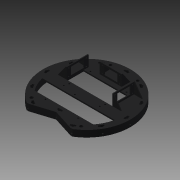
# Autodesk Inventor part: Middle Plate
Saved by Autodesk Inventor 2015 (Build 190159000, 159)
## iProperties
Created: 2015-10-10
Part Number: Middle Plate
Material: ABS Plastic
Document SubType Name: Modeling
Designer: James
Density: 1.06 g/cm^3
Appearance: Smooth - White
Mass: 170.874 g
Surface Area: 729.36 cm^2
Volume: 161.202 cm^3
Author: James
Autodesk Inventor part; units mm, degrees
ref_plane "YZ Plane" through (0, 0, 0) normal (1, 0, 0) x (0, 1, 0)
ref_plane "XZ Plane" through (0, 0, 0) normal (0, 1, 0) x (-1, 0, 0)
ref_plane "XY Plane" through (0, 0, 0) normal (0, 0, 1) x (1, 0, 0)
sketch "Sketch1" plane through (0, 0, 0) normal (0, 1, 0) x (-1, 0, 0)
  line L0 (70, 0) -> (70, 48.2183)
  line L1 (70, 0) -> (70, -48.2183)
  arc A0 (70, 48.2183) -> (70, -48.2183) centre (0, 0) ccw
  arc A1 (85, 52.6783) -> (85, -52.6783) centre (0, 0) ccw
  line L2 (85, -52.6783) -> (85, -47.6783)
  line L3 (85, 52.6783) -> (85, 47.6783)
  line L4 (85, -47.6783) -> (70, 0)
  line L5 (70, 0) -> (85, 47.6783)
  dimension "d332" = 5
  dimension "d333" = 5
  constraints: 12 end point, 4 point on circle, 2 centre point, 1 coincident, 1 point on line, 1 vertical
  measures "d332" distance of L2.start L2.end
  measures "d333" distance of L3.start L3.end
extrude "Extrusion1" add sketch "Sketch1" along normal blind 15
sketch "Sketch2" plane through (0, 15, 0) normal (0, 1, 0) x (1, 0, 0)
  line L0 (0, 0) -> (71.6532, -61.1111) construction
  line L1 (0, 0) -> (88.2332, 32.9188) construction
  line L2 (0, 0) -> (71.6532, 61.1111) construction
  circle A0 centre (85.6755, -31.1833) radius 3
  circle A1 centre (85.6755, 31.1833) radius 3
  circle A2 centre (-69.5802, -56.8899) radius 3.5
  circle A3 centre (-69.5802, 56.8899) radius 3.5
  dimension "d409" = 20
  dimension "d495" = 7
  dimension "d496" = 7
  constraints: 6 end point, 4 centre point, 2 coincident
  measures "d409" angle of L1 L2
  measures "d495" diameter of A2
  measures "d496" diameter of A3
extrude "Extrusion2" cut sketch "Sketch2" against normal blind 15
sketch "Sketch3" plane through (0, 15, 0) normal (0, 1, 0) x (1, 0, 0)
  line L0 (89.1, -5.2) -> (89.1, 5.2)
  arc A0 (93.2, -2.6833) -> (93.2, 2.6833) centre (92.1, 0) ccw
  line L1 (89.1, -5.2) -> (93.2, -5.2)
  line L2 (93.2, -2.6833) -> (93.2, -5.2)
  line L3 (93.2, 5.2) -> (93.2, 2.6833)
  line L4 (89.1, 5.2) -> (93.2, 5.2)
  line L5 (79.7629, 40.0467) -> (83.3136, 42.0967)
  line L6 (82.0552, 44.2762) -> (83.3136, 42.0967)
  arc A1 (82.0552, 44.2762) -> (79.3719, 48.9238) centre (79.7609, 46.05) ccw
  line L7 (78.1136, 51.1033) -> (79.3719, 48.9238)
  line L8 (74.5629, 49.0533) -> (78.1136, 51.1033)
  line L9 (79.7629, 40.0467) -> (74.5629, 49.0533)
  line L10 (49.0533, 74.5629) -> (51.1033, 78.1136)
  line L11 (48.9238, 79.3719) -> (51.1033, 78.1136)
  arc A2 (48.9238, 79.3719) -> (44.2762, 82.0552) centre (46.05, 79.7609) ccw
  line L12 (42.0967, 83.3136) -> (44.2762, 82.0552)
  line L13 (40.0467, 79.7629) -> (42.0967, 83.3136)
  line L14 (49.0533, 74.5629) -> (40.0467, 79.7629)
  line L15 (5.2, 89.1) -> (5.2, 93.2)
  line L16 (2.6833, 93.2) -> (5.2, 93.2)
  arc A3 (2.6833, 93.2) -> (-2.6833, 93.2) centre (0, 92.1) ccw
  line L17 (-5.2, 93.2) -> (-2.6833, 93.2)
  line L18 (-5.2, 89.1) -> (-5.2, 93.2)
  line L19 (5.2, 89.1) -> (-5.2, 89.1)
  line L20 (-40.0467, 79.7629) -> (-42.0967, 83.3136)
  line L21 (-44.2762, 82.0552) -> (-42.0967, 83.3136)
  arc A4 (-44.2762, 82.0552) -> (-48.9238, 79.3719) centre (-46.05, 79.7609) ccw
  line L22 (-51.1033, 78.1136) -> (-48.9238, 79.3719)
  line L23 (-49.0533, 74.5629) -> (-51.1033, 78.1136)
  line L24 (-40.0467, 79.7629) -> (-49.0533, 74.5629)
  line L25 (-72.5629, 49.0533) -> (-76.1136, 51.1033)
  line L26 (-77.3719, 48.9238) -> (-76.1136, 51.1033)
  arc A5 (-77.3719, 48.9238) -> (-80.0552, 44.2762) centre (-77.7609, 46.05) ccw
  line L27 (-81.3136, 42.0967) -> (-80.0552, 44.2762)
  line L28 (-77.7629, 40.0467) -> (-81.3136, 42.0967)
  line L29 (-72.5629, 49.0533) -> (-77.7629, 40.0467)
  line L30 (-59.1, 5.2) -> (-63.2, 5.2)
  line L31 (-63.2, 2.6833) -> (-63.2, 5.2)
  arc A6 (-63.2, 2.6833) -> (-63.2, -2.6833) centre (-62.1, 0) ccw
  line L32 (-63.2, -5.2) -> (-63.2, -2.6833)
  line L33 (-59.1, -5.2) -> (-63.2, -5.2)
  line L34 (-59.1, 5.2) -> (-59.1, -5.2)
  line L35 (-77.7629, -40.0467) -> (-81.3136, -42.0967)
  line L36 (-80.0552, -44.2762) -> (-81.3136, -42.0967)
  arc A7 (-80.0552, -44.2762) -> (-77.3719, -48.9238) centre (-77.7609, -46.05) ccw
  line L37 (-76.1136, -51.1033) -> (-77.3719, -48.9238)
  line L38 (-72.5629, -49.0533) -> (-76.1136, -51.1033)
  line L39 (-77.7629, -40.0467) -> (-72.5629, -49.0533)
  line L40 (-49.0533, -74.5629) -> (-51.1033, -78.1136)
  line L41 (-48.9238, -79.3719) -> (-51.1033, -78.1136)
  arc A8 (-48.9238, -79.3719) -> (-44.2762, -82.0552) centre (-46.05, -79.7609) ccw
  line L42 (-42.0967, -83.3136) -> (-44.2762, -82.0552)
  line L43 (-40.0467, -79.7629) -> (-42.0967, -83.3136)
  line L44 (-49.0533, -74.5629) -> (-40.0467, -79.7629)
  line L45 (-5.2, -89.1) -> (-5.2, -93.2)
  line L46 (-2.6833, -93.2) -> (-5.2, -93.2)
  arc A9 (-2.6833, -93.2) -> (2.6833, -93.2) centre (0, -92.1) ccw
  line L47 (5.2, -93.2) -> (2.6833, -93.2)
  line L48 (5.2, -89.1) -> (5.2, -93.2)
  line L49 (-5.2, -89.1) -> (5.2, -89.1)
  line L50 (40.0467, -79.7629) -> (42.0967, -83.3136)
  line L51 (44.2762, -82.0552) -> (42.0967, -83.3136)
  arc A10 (44.2762, -82.0552) -> (48.9238, -79.3719) centre (46.05, -79.7609) ccw
  line L52 (51.1033, -78.1136) -> (48.9238, -79.3719)
  line L53 (49.0533, -74.5629) -> (51.1033, -78.1136)
  line L54 (40.0467, -79.7629) -> (49.0533, -74.5629)
  line L55 (74.5629, -49.0533) -> (78.1136, -51.1033)
  line L56 (79.3719, -48.9238) -> (78.1136, -51.1033)
  arc A11 (79.3719, -48.9238) -> (82.0552, -44.2762) centre (79.7609, -46.05) ccw
  line L57 (83.3136, -42.0967) -> (82.0552, -44.2762)
  line L58 (79.7629, -40.0467) -> (83.3136, -42.0967)
  line L59 (74.5629, -49.0533) -> (79.7629, -40.0467)
  point P0 (0, 0)
  point P1 (92.1, 0)
  point P2 (79.7609, 46.05)
  point P3 (46.05, 79.7609)
  point P4 (0, 92.1)
  point P5 (-46.05, 79.7609)
  point P6 (-77.7609, 46.05)
  point P7 (-62.1, 0)
  point P8 (-77.7609, -46.05)
  point P9 (-46.05, -79.7609)
  point P10 (0, -92.1)
  point P11 (46.05, -79.7609)
  point P12 (79.7609, -46.05)
  point P13 (-70, 0)
  dimension "d118" = 270
  dimension "d123" = 255
  dimension "d347" = 360
  constraints: 120 end point, 24 point on circle, 12 centre point, 12 coincident, 123 other
sketch "Sketch8" plane through (0, 0, 0) normal (0, -1, 0) x (1, 0, 0)
  line L0 (-70, 48.2183) -> (-70, -48.2183)
  arc A0 (-70, -48.2183) -> (-70, 48.2183) centre (0, 0) ccw projected
  line L1 (-52, -48.2183) -> (-52, -67.2384)
  arc A1 (-57, 63.0555) -> (-70, 48.2183) centre (0, 0) ccw
  arc A2 (-70, -48.2183) -> (-52, -67.2384) centre (0, 0) ccw
  line L2 (-52, -48.2183) -> (-52, 67.2384)
  arc A3 (-70, -48.2183) -> (-70, 48.2183) centre (0, 0) ccw projected
  line L3 (-52, -48.2183) -> (63.4566, -48.2183) construction
  dimension "d54" = 18
  dimension "d336" = 90
  constraints: 8 end point, 7 point on circle, 2 centre point, 2 coincident, 2 vertical, 1 horizontal, 1 perpendicular
  measures "d54" distance of L0.end L1.start
  measures "d336" angle of L3 L2
extrude "Extrusion8" add sketch "Sketch8" against normal blind 15 contours A0 L2 L1 L0
sketch "Sketch9" plane through (0, 15, 0) normal (0, 1, 0) x (1, 0, 0)
  circle A0 centre (-8.778, -38.7103) radius 1.6079
  circle A1 centre (-62, -39.9697) radius 1.6079
  circle A2 centre (-62, 34.9127) radius 1.6079
  circle A3 centre (-8.7782, 43.7683) radius 1.6079
  line L0 (-57, 67.2384) -> (-57, -67.2384) projected
  line L1 (-18.7782, -41.2393) -> (-18.7782, -82.8998)
  arc A4 (-52, -67.2384) -> (-52, 67.2384) centre (0, 0) ccw projected
  line L2 (-18.7782, -41.2393) -> (-18.7782, 82.8998)
  line L3 (6.2218, 0) -> (6.2218, -84.772)
  line L4 (6.2218, 84.772) -> (6.2218, 0)
  arc A5 (-18.7782, -82.8998) -> (6.2218, -84.772) centre (0, 0) ccw
  arc A6 (6.2218, 84.772) -> (-18.7782, 82.8998) centre (0, 0) ccw
  circle A7 centre (-13.8564, 13.3202) radius 1.6079
  circle A8 centre (1.2218, -41.2393) radius 1.65
  circle A9 centre (1.2218, 41.2393) radius 1.65
  circle A10 centre (1.2218, -41.2393) radius 1.65
  point P0 (-8.7782, -84.5455)
  point P1 (-8.7782, 84.5455)
  dimension "d67" = 10.315
  dimension "d434" = 3.3
  dimension "d435" = 3.3
  constraints: 10 centre point, 10 point on circle, 8 end point, 2 coincident, 2 point on line, 1 collinear, 1 vertical alignment
  measures "d67" distance of A0.centre L1.start
  measures "d434" diameter of A8
  measures "d435" diameter of A9
sketch "Sketch10" plane through (0, 15, 0) normal (0, 1, 0) x (1, 0, 0)
  circle A0 centre (-57, -37.4412) radius 1.65
  circle A1 centre (-57, 37.4412) radius 1.65
  point P0 (0, 0)
  dimension "d71" = 3.3
  dimension "d72" = 3.3
  constraints: 2 centre point
  measures "d71" diameter of A0
  measures "d72" diameter of A1
extrude "Extrusion10" cut sketch "Sketch10" against normal blind 10
sketch "Sketch34" plane through (0, 15, 0) normal (0, 1, 0) x (1, 0, 0)
  arc A0 (-52, -67.2384) -> (-52, 67.2384) centre (0, 0) ccw projected
  line L0 (45, 0) -> (45, -72.111)
  line L1 (45, 0) -> (45, 72.111)
  arc A1 (45, -72.111) -> (45, 72.111) centre (0, 0) ccw
  point P0 (6.2218, 84.772)
  point P1 (6.2218, -84.772)
  constraints: 4 end point, 4 point on circle, 1 centre point, 1 coincident, 1 point on line
extrude "Extrusion34" add sketch "Sketch34" against normal blind 3
sketch "Sketch35" plane through (0, 15, 0) normal (0, 1, 0) x (1, 0, 0)
  arc A0 (45, 72.111) -> (-52, 67.2384) centre (0, 0) ccw projected
  line L0 (-52, -67.2384) -> (-52, 67.2384) projected
  circle A1 centre (-57, -37.4412) radius 1.65 projected
  circle A2 centre (-57, 37.4412) radius 1.65 projected
  line L1 (45, 72.111) -> (45, -72.111) projected
  arc A3 (-85, -52.6783) -> (-85, 52.6783) centre (0, 0) ccw projected
  circle A4 centre (50, -41.2393) radius 1.65
  circle A5 centre (50, 41.4252) radius 1.65
  line L2 (-85, 52.6783) -> (-85, 47.6783) projected
  line L3 (-85, -47.6783) -> (-85, -52.6783) projected
  line L4 (-70, 0) -> (-85, -47.6783) projected
  line L5 (-85, 47.6783) -> (-70, 0) projected
  arc A6 (-52, -67.2384) -> (45, -72.111) centre (0, 0) ccw projected
  dimension "d223" = 3.3
  dimension "d224" = 3.3
  constraints: 2 centre point
  measures "d223" diameter of A4
  measures "d224" diameter of A5
extrude "Extrusion35" cut sketch "Sketch35" against normal blind 5 contours A4 | A5
fillet "Fillet1" radius 2 4 edges at (-85, 7.5, -52.6783) (-85, 7.5, -47.6783) (-85, 7.5, 47.6783) (-85, 7.5, 52.6783)
fillet "Fillet2" radius 2 1 edges at (-70, 7.5, 0)
extrude "Extrusion49" cut sketch "Sketch3" against normal blind 13
sketch "Sketch51" plane through (-59.1, 15, -5.2) normal (-1, 0, 0) x (0, 0, 1)
  line L0 (0, 0) -> (10.4, 0) projected
  line L1 (5.2, 0) -> (5.2, -9.7)
  line L2 (5.2, 0) -> (14.9, 0) construction
  circle A0 centre (5.2, -9.6872) radius 1.5
  point P0 (5.2, -15)
  dimension "d352" = 9.7
  dimension "d353" = 90
  dimension "d354" = 3
  constraints: 4 end point, 1 centre point, 1 horizontal, 1 midpoint, 1 perpendicular, 1 point on line, 1 vertical
  measures "d352" distance of L1.start L1.end
  measures "d353" angle of L1 L2
  measures "d354" diameter of A0
extrude "Extrusion50" cut sketch "Sketch51" along normal blind 22
sketch "Sketch52" plane through (-72.5629, 2, -49.0533) normal (-0.8660254, 0, -0.5) x (-0.5, 0, 0.8660254)
  line L0 (0, 13) -> (10.4, 13) projected
  line L1 (5.2, 13) -> (5.2, 3.3)
  line L2 (5.2, 13) -> (14.9, 13) construction
  circle A0 centre (5.2, 3.3) radius 1.5
  point P0 (6.2, -2)
  dimension "d357" = 9.7
  dimension "d358" = 90
  dimension "d359" = 3
  constraints: 4 end point, 1 centre point, 1 coincident, 1 horizontal, 1 midpoint, 1 perpendicular, 1 vertical
  measures "d357" distance of L1.start L1.end
  measures "d358" angle of L1 L2
  measures "d359" diameter of A0
extrude "Extrusion51" cut sketch "Sketch52" along normal blind 22
sketch "Sketch53" plane through (-40.0467, 2, -79.7629) normal (-0.5, 0, -0.8660254) x (-0.8660254, 0, 0.5)
  line L0 (0, 13) -> (10.4, 13) projected
  line L1 (5.2, 13) -> (5.2, 3.3)
  circle A0 centre (5.2, 3.3) radius 1.5
  point P0 (5.2, -2)
  dimension "d362" = 9.7
  dimension "d363" = 3
  constraints: 2 end point, 1 centre point, 1 coincident, 1 midpoint, 1 vertical
  measures "d362" distance of L1.start L1.end
  measures "d363" diameter of A0
extrude "Extrusion52" cut sketch "Sketch53" along normal blind 22
sketch "Sketch54" plane through (5.2, 15, -89.1) normal (0, 0, -1) x (-1, 0, 0)
  line L0 (0, 0) -> (10.4, 0) projected
  line L1 (5.2, 0) -> (5.2, -9.7)
  line L2 (5.2, 0) -> (14.9, 0) construction
  circle A0 centre (5.2, -9.7) radius 1.5
  point P0 (5.2, -15)
  dimension "d366" = 9.7
  dimension "d367" = 90
  dimension "d368" = 3
  constraints: 4 end point, 1 centre point, 1 coincident, 1 horizontal, 1 midpoint, 1 perpendicular, 1 vertical
  measures "d366" distance of L1.start L1.end
  measures "d367" angle of L1 L2
  measures "d368" diameter of A0
extrude "Extrusion53" cut sketch "Sketch54" along normal blind 22
sketch "Sketch55" plane through (49.0533, 2, -74.5629) normal (0.5, 0, -0.8660254) x (-0.8660254, 0, -0.5)
  line L0 (0, 13) -> (10.4, 13) projected
  line L1 (5.2, 13) -> (5.2, 3.3)
  circle A0 centre (5.2, 3.3) radius 1.5
  point P0 (5.2, -2)
  dimension "d371" = 9.7
  dimension "d372" = 3
  constraints: 2 end point, 1 centre point, 1 coincident, 1 midpoint, 1 vertical
  measures "d371" distance of L1.start L1.end
  measures "d372" diameter of A0
extrude "Extrusion54" cut sketch "Sketch55" along normal blind 22
sketch "Sketch56" plane through (79.7629, 2, -40.0467) normal (0.8660254, 0, -0.5) x (-0.5, 0, -0.8660254)
  line L0 (0, 13) -> (10.4, 13) projected
  line L1 (5.2, 13) -> (5.2, 3.3)
  circle A0 centre (5.2, 3.3) radius 1.5
  point P0 (5.2, -2)
  dimension "d375" = 9.7
  dimension "d376" = 3
  constraints: 2 end point, 1 centre point, 1 coincident, 1 midpoint, 1 vertical
  measures "d375" distance of L1.start L1.end
  measures "d376" diameter of A0
extrude "Extrusion55" cut sketch "Sketch56" along normal blind 22
sketch "Sketch57" plane through (89.1, 15, 5.2) normal (1, 0, 0) x (0, 0, -1)
  line L0 (0, 0) -> (10.4, 0) projected
  line L1 (5.2, 0) -> (5.2, -9.7)
  circle A0 centre (5.2, -9.7) radius 1.5
  point P0 (5.2, -15)
  dimension "d379" = 9.7
  dimension "d380" = 3
  constraints: 2 end point, 1 centre point, 1 coincident, 1 midpoint, 1 vertical
  measures "d379" distance of L1.start L1.end
  measures "d380" diameter of A0
extrude "Extrusion56" cut sketch "Sketch57" along normal blind 22
sketch "Sketch58" plane through (74.5629, 2, 49.0533) normal (0.8660254, 0, 0.5) x (0.5, 0, -0.8660254)
  line L0 (0, 13) -> (10.4, 13) projected
  line L1 (5.2, 13) -> (5.2, 3.3)
  circle A0 centre (5.2, 3.3) radius 1.5
  point P0 (5.2, -2)
  dimension "d383" = 9.7
  dimension "d384" = 3
  constraints: 2 end point, 1 centre point, 1 coincident, 1 midpoint, 1 vertical
  measures "d383" distance of L1.start L1.end
  measures "d384" diameter of A0
extrude "Extrusion57" cut sketch "Sketch58" along normal blind 22
sketch "Sketch59" plane through (40.0467, 2, 79.7629) normal (0.5, 0, 0.8660254) x (0.8660254, 0, -0.5)
  line L0 (0, 13) -> (10.4, 13) projected
  line L1 (5.2, 13) -> (5.2, 3.3)
  circle A0 centre (5.2, 3.3) radius 1.5
  point P0 (5.2, -2)
  dimension "d387" = 9.7
  dimension "d388" = 3
  constraints: 2 end point, 1 centre point, 1 coincident, 1 midpoint, 1 vertical
  measures "d387" distance of L1.start L1.end
  measures "d388" diameter of A0
extrude "Extrusion58" cut sketch "Sketch59" along normal blind 22
sketch "Sketch60" plane through (-5.2, 15, 89.1) normal (0, 0, 1) x (1, 0, 0)
  line L0 (0, 0) -> (10.4, 0) projected
  line L1 (5.2, 0) -> (5.2, -9.7)
  line L2 (5.2, 0) -> (14.9, 0) construction
  circle A0 centre (5.2, -9.7) radius 1.5
  point P0 (5.2, -15)
  dimension "d391" = 9.7
  dimension "d392" = 90
  dimension "d393" = 3
  constraints: 4 end point, 1 centre point, 1 coincident, 1 horizontal, 1 midpoint, 1 perpendicular, 1 vertical
  measures "d391" distance of L1.start L1.end
  measures "d392" angle of L1 L2
  measures "d393" diameter of A0
extrude "Extrusion59" cut sketch "Sketch60" along normal blind 22
sketch "Sketch61" plane through (-49.0533, 2, 74.5629) normal (-0.5, 0, 0.8660254) x (0.8660254, 0, 0.5)
  line L0 (0, 13) -> (10.4, 13) projected
  line L1 (5.2, 13) -> (5.2, 3.3)
  line L2 (5.2, 13) -> (14.9, 13) construction
  circle A0 centre (5.2, 3.3) radius 1.5
  point P0 (5.2, -2)
  dimension "d396" = 9.7
  dimension "d397" = 90
  dimension "d398" = 3
  constraints: 4 end point, 1 centre point, 1 coincident, 1 horizontal, 1 midpoint, 1 perpendicular, 1 vertical
  measures "d396" distance of L1.start L1.end
  measures "d397" angle of L1 L2
  measures "d398" diameter of A0
extrude "Extrusion60" cut sketch "Sketch61" along normal blind 22
sketch "Sketch62" plane through (-77.7629, 2, 40.0467) normal (-0.8660254, 0, 0.5) x (0.5, 0, 0.8660254)
  line L0 (0, 13) -> (10.4, 13) projected
  line L1 (5.2, 13) -> (5.2, 3.3)
  circle A0 centre (5.2, 3.3) radius 1.5
  point P0 (4.2, -2)
  dimension "d401" = 9.7
  dimension "d402" = 3
  constraints: 2 end point, 1 centre point, 1 coincident, 1 midpoint, 1 vertical
  measures "d401" distance of L1.start L1.end
  measures "d402" diameter of A0
extrude "Extrusion61" cut sketch "Sketch62" along normal blind 22
sketch "Sketch63" plane through (0, 0, 0) normal (0, -1, 0) x (1, 0, 0)
  line L0 (44.2762, 82.0552) -> (42.0967, 83.3136) projected
  line L1 (42.0967, 83.3136) -> (40.0467, 79.7629) projected
  line L2 (40.0467, 79.7629) -> (49.0533, 74.5629) projected
  line L3 (49.0533, 74.5629) -> (51.1033, 78.1136) projected
  line L4 (51.1033, 78.1136) -> (48.9238, 79.3719) projected
  arc A0 (48.9238, 79.3719) -> (44.2762, 82.0552) centre (46.05, 79.7609) ccw projected
  line L5 (-48.9238, 79.3719) -> (-51.1033, 78.1136) projected
  line L6 (-51.1033, 78.1136) -> (-49.0533, 74.5629) projected
  line L7 (-49.0533, 74.5629) -> (-40.0467, 79.7629) projected
  line L8 (-40.0467, 79.7629) -> (-42.0967, 83.3136) projected
  line L9 (-42.0967, 83.3136) -> (-44.2762, 82.0552) projected
  arc A1 (-44.2762, 82.0552) -> (-48.9238, 79.3719) centre (-46.05, 79.7609) ccw projected
  line L10 (-63.2, -2.6833) -> (-63.2, -5.2) projected
  line L11 (-63.2, -5.2) -> (-59.1, -5.2) projected
  line L12 (-59.1, -5.2) -> (-59.1, 5.2) projected
  line L13 (-59.1, 5.2) -> (-63.2, 5.2) projected
  line L14 (-63.2, 5.2) -> (-63.2, 2.6833) projected
  arc A2 (-63.2, 2.6833) -> (-63.2, -2.6833) centre (-62.1, 0) ccw projected
  line L15 (-44.2762, -82.0552) -> (-42.0967, -83.3136) projected
  line L16 (-42.0967, -83.3136) -> (-40.0467, -79.7629) projected
  line L17 (-40.0467, -79.7629) -> (-49.0533, -74.5629) projected
  line L18 (-49.0533, -74.5629) -> (-51.1033, -78.1136) projected
  line L19 (-51.1033, -78.1136) -> (-48.9238, -79.3719) projected
  arc A3 (-48.9238, -79.3719) -> (-44.2762, -82.0552) centre (-46.05, -79.7609) ccw projected
  line L20 (48.9238, -79.3719) -> (51.1033, -78.1136) projected
  line L21 (51.1033, -78.1136) -> (49.0533, -74.5629) projected
  line L22 (49.0533, -74.5629) -> (40.0467, -79.7629) projected
  line L23 (40.0467, -79.7629) -> (42.0967, -83.3136) projected
  line L24 (42.0967, -83.3136) -> (44.2762, -82.0552) projected
  arc A4 (44.2762, -82.0552) -> (48.9238, -79.3719) centre (46.05, -79.7609) ccw projected
  line L25 (93.2, 2.6833) -> (93.2, 5.2) projected
  line L26 (93.2, 5.2) -> (89.1, 5.2) projected
  line L27 (89.1, 5.2) -> (89.1, -5.2) projected
  line L28 (89.1, -5.2) -> (93.2, -5.2) projected
  line L29 (93.2, -5.2) -> (93.2, -2.6833) projected
  arc A5 (93.2, -2.6833) -> (93.2, 2.6833) centre (92.1, 0) ccw projected
  line L30 (82.0552, -44.2762) -> (83.3136, -42.0967) projected
  line L31 (83.3136, -42.0967) -> (79.7629, -40.0467) projected
  line L32 (79.7629, -40.0467) -> (74.5629, -49.0533) projected
  line L33 (74.5629, -49.0533) -> (78.1136, -51.1033) projected
  line L34 (78.1136, -51.1033) -> (79.3719, -48.9238) projected
  arc A6 (79.3719, -48.9238) -> (82.0552, -44.2762) centre (79.7609, -46.05) ccw projected
  line L35 (2.6833, -93.2) -> (5.2, -93.2) projected
  line L36 (5.2, -93.2) -> (5.2, -89.1) projected
  line L37 (5.2, -89.1) -> (-5.2, -89.1) projected
  line L38 (-5.2, -89.1) -> (-5.2, -93.2) projected
  line L39 (-5.2, -93.2) -> (-2.6833, -93.2) projected
  arc A7 (-2.6833, -93.2) -> (2.6833, -93.2) centre (0, -92.1) ccw projected
  line L40 (-77.3719, -48.9238) -> (-76.1136, -51.1033) projected
  line L41 (-76.1136, -51.1033) -> (-72.5629, -49.0533) projected
  line L42 (-72.5629, -49.0533) -> (-77.7629, -40.0467) projected
  line L43 (-77.7629, -40.0467) -> (-81.3136, -42.0967) projected
  line L44 (-81.3136, -42.0967) -> (-80.0552, -44.2762) projected
  arc A8 (-80.0552, -44.2762) -> (-77.3719, -48.9238) centre (-77.7609, -46.05) ccw projected
  line L45 (-80.0552, 44.2762) -> (-81.3136, 42.0967) projected
  line L46 (-81.3136, 42.0967) -> (-77.7629, 40.0467) projected
  line L47 (-77.7629, 40.0467) -> (-72.5629, 49.0533) projected
  line L48 (-72.5629, 49.0533) -> (-76.1136, 51.1033) projected
  line L49 (-76.1136, 51.1033) -> (-77.3719, 48.9238) projected
  arc A9 (-77.3719, 48.9238) -> (-80.0552, 44.2762) centre (-77.7609, 46.05) ccw projected
  line L50 (-2.6833, 93.2) -> (-5.2, 93.2) projected
  line L51 (-5.2, 93.2) -> (-5.2, 89.1) projected
  line L52 (-5.2, 89.1) -> (5.2, 89.1) projected
  line L53 (5.2, 89.1) -> (5.2, 93.2) projected
  line L54 (5.2, 93.2) -> (2.6833, 93.2) projected
  arc A10 (2.6833, 93.2) -> (-2.6833, 93.2) centre (0, 92.1) ccw projected
  line L55 (79.3719, 48.9238) -> (78.1136, 51.1033) projected
  line L56 (78.1136, 51.1033) -> (74.5629, 49.0533) projected
  line L57 (74.5629, 49.0533) -> (79.7629, 40.0467) projected
  line L58 (79.7629, 40.0467) -> (83.3136, 42.0967) projected
  line L59 (83.3136, 42.0967) -> (82.0552, 44.2762) projected
  arc A11 (82.0552, 44.2762) -> (79.3719, 48.9238) centre (79.7609, 46.05) ccw projected
  arc A12 (-84.6939, 53.169) -> (-85, 52.1057) centre (-83, 52.1057) ccw projected
  arc A13 (-84.6939, -53.169) -> (-84.6939, 53.169) centre (0, 0) ccw projected
  arc A14 (-85, -52.1057) -> (-84.6939, -53.169) centre (-83, -52.1057) ccw projected
  line L60 (-85, -52.1057) -> (-85, -47.9855) projected
  arc A15 (-84.9078, -47.3852) -> (-85, -47.9855) centre (-83, -47.9855) ccw projected
  line L61 (-84.9078, -47.3852) -> (-70.1888, -0.6002) projected
  arc A16 (-70.1888, -0.6002) -> (-70.1888, 0.6002) centre (-72.0966, 0) ccw projected
  line L62 (-70.1888, 0.6002) -> (-84.9078, 47.3852) projected
  arc A17 (-85, 47.9855) -> (-84.9078, 47.3852) centre (-83, 47.9855) ccw projected
  line L63 (-85, 47.9855) -> (-85, 52.1057) projected
  circle A18 centre (50, 41.2393) radius 1.65 projected
  circle A19 centre (50, -41.4252) radius 1.65 projected
  arc A20 (-52, -67.2384) -> (45, -72.111) centre (0, 0) ccw projected
  line L64 (-52, 67.2384) -> (-52, -67.2384) projected
  circle A21 centre (-57, 37.4412) radius 1.65 projected
  circle A22 centre (-57, -37.4412) radius 1.65 projected
  circle A23 centre (85.6755, -31.1833) radius 3 projected
  circle A24 centre (85.6755, 31.1833) radius 3 projected
  line L65 (45, -72.111) -> (45, 72.111) projected
  circle A25 centre (-57, -37.4412) radius 1.65 projected
  line L66 (-52, -67.2384) -> (-52, 67.2384) projected
  line L67 (-52, 67.2384) -> (-52, -67.2384) projected
  line L68 (-52, -47.4412) -> (-52, -27.4412)
  line L69 (-52, 27.4412) -> (-52, 47.4412)
  line L70 (-64, -37.4412) -> (-49.0294, -37.4412) construction
  line L71 (-64, -37.4412) -> (-49.0294, -37.4412) construction
  line L72 (-52, 49.4412) -> (-52, 25.4412)
  line L73 (-52, -25.4412) -> (-52, -49.4412)
  arc A26 (45, 72.111) -> (-52, 67.2384) centre (0, 0) ccw projected
  arc A27 (-52, 67.2384) -> (-70.4899, 47.4992) centre (0, 0) ccw
  line L74 (-52, 0) -> (-55, 0)
  line L75 (-55.2236, 0.6503) -> (-70.7227, 45.7313)
  arc A28 (-70.4899, -47.4992) -> (-52, -67.2384) centre (0, 0) ccw
  line L76 (-55.2236, -0.6503) -> (-70.7227, -45.7313)
  arc A29 (-70.4899, 47.4992) -> (-70.7227, 45.7313) centre (-68.8313, 46.3816) ccw
  arc A30 (-55.2236, -0.6503) -> (-55.2236, 0.6503) centre (-57.1149, 0) ccw
  arc A31 (-70.7227, -45.7313) -> (-70.4899, -47.4992) centre (-68.8313, -46.3816) ccw
  point P0 (-71.0441, 46.6662)
  point P1 (-71.0441, -46.6662)
  dimension "d411" = 7
  dimension "d442" = 3
  dimension "d443" = 2
  constraints: 18 end point, 12 point on circle, 12 point on line, 6 tangent, 5 centre point, 4 collinear, 3 horizontal, 2 equal radius, 1 coincident, 1 midpoint
  measures "d411" distance of A25.centre L70.start
  measures "d442" distance of L74.start L74.end
  measures "d443" radius of A29
extrude "Extrusion62" cut sketch "Sketch63" against normal blind 12 contours L64 A26 L65 A20 | A28 A31 L76 A30 L75 A29 A27 L64 | A21 | A22
extrude "Extrusion65" add sketch "Sketch9" against normal blind 3 contours L2 A4 L4 L3 L1
sketch "Sketch64" plane through (0, 15, 0) normal (0, 1, 0) x (1, 0, 0)
  line L0 (45, -72.111) -> (45, -52.111)
  line L1 (45, -72.111) -> (45, 72.111) projected
  line L2 (45, -52.111) -> (6.2218, -52.111)
  line L3 (6.2218, -84.772) -> (6.2218, 84.772) projected
  line L4 (6.2218, -72.111) -> (6.2218, -52.111)
  arc A0 (6.2218, -84.772) -> (45, -72.111) centre (0, 0) ccw
  line L5 (6.2218, -84.772) -> (6.2218, -52.111)
  line L6 (6.2218, 84.772) -> (6.2218, -84.772) projected
  dimension "d444" = 20
  constraints: 8 end point, 3 point on line, 2 collinear, 2 point on circle, 1 centre point, 1 coincident, 1 perpendicular
  measures "d444" distance of L0.start L0.end
extrude "Extrusion66" add sketch "Sketch64" against normal blind 3
sketch "Sketch65" plane through (0, 15, 0) normal (0, 1, 0) x (1, 0, 0)
  line L0 (6.2218, -52.111) -> (56.2218, -52.111)
  line L1 (56.2218, -52.111) -> (56.2218, -54.111)
  line L2 (6.2218, -54.111) -> (6.2218, -52.111)
  line L3 (6.2218, -54.111) -> (6.2218, -72.111)
  line L4 (6.2218, -72.111) -> (8.2218, -72.111)
  line L5 (8.2218, -72.111) -> (8.2218, -54.111)
  line L6 (56.2218, -54.111) -> (56.2218, -72.111)
  line L7 (56.2218, -72.111) -> (54.2218, -72.111)
  line L8 (54.2218, -72.111) -> (54.2218, -54.111)
  line L9 (8.2218, -54.111) -> (54.2218, -54.111)
  point P0 (0, 0)
  dimension "d447" = 50
  dimension "d448" = 2
  dimension "d451" = 2
  dimension "d452" = 2
  constraints: 20 end point, 4 perpendicular, 3 parallel, 2 horizontal, 1 point on line
  measures "d447" distance of L0.start L0.end
  measures "d448" distance of L0.end L1.end
  measures "d451" distance of L4.end L3.end
  measures "d452" distance of L6.end L7.end
extrude "Extrusion67" add sketch "Sketch65" along normal blind 25
chamfer "Chamfer2" distance 18 distance2 25 1 edges at (55.2218, 40, 72.111) measured on face at (23.5551, 40, 52.7777)
chamfer "Chamfer3" distance 18 distance2 25 1 edges at (7.2218, 40, 72.111) measured on face at (23.5551, 40, 52.7777)
sketch "Sketch67" plane through (8.2218, 15, 54.111) normal (0, 0, 1) x (1, 0, 0)
  point P0 (-8.2218, -15)
sketch "Sketch68" plane through (8.2218, 15, 54.111) normal (0, 0, 1) x (1, 0, 0)
  line L0 (0, 0) -> (0, 25) projected
  line L1 (48, 25) -> (-2, 25) projected
  circle A0 centre (3, 21) radius 1.25
  circle A1 centre (3, 4) radius 1.25
  circle A2 centre (43, 4) radius 1.25
  circle A3 centre (43, 21) radius 1.25
  line L2 (8, 4) -> (8, 21)
  line L3 (8, 21) -> (38, 21)
  line L4 (38, 21) -> (38, 4)
  line L5 (38, 4) -> (8, 4)
  point P0 (-8.2218, -15)
  dimension "d467" = 2.5
  dimension "d469" = 2.5
  dimension "d470" = 2.5
  dimension "d471" = 5
  dimension "d472" = 30
  constraints: 8 end point, 4 centre point, 3 perpendicular
  measures "d467" diameter of A0
  measures "d469" diameter of A2
  measures "d470" diameter of A3
  measures "d471" distance of A1.centre L2.start
  measures "d472" distance of L2.end L3.end
extrude "Extrusion68" cut sketch "Sketch68" against normal blind 25
mirror "Mirror1" about plane through (0, 0, 0) normal (0, 0, 1) of "Extrusion67", "Extrusion66", "Chamfer2", "Chamfer3", "Extrusion68"
sketch "Sketch69" plane through (0, 15, 0) normal (0, 1, 0) x (1, 0, 0)
  line L0 (55, -25) -> (55, 25)
  line L1 (55, 25) -> (57, 25)
  line L2 (57, -25) -> (55, -25)
  line L3 (57, -25) -> (75, -25)
  line L4 (75, -25) -> (75, -23)
  line L5 (75, -23) -> (57, -23)
  line L6 (57, 25) -> (75, 25)
  line L7 (75, 23) -> (57, 23)
  line L8 (57, -23) -> (57, 23)
  line L9 (45, 52.111) -> (45, -52.111) projected
  line L10 (75, 25) -> (75, 23)
  point P0 (0, 0)
  dimension "d475" = 50
  dimension "d476" = 2
  dimension "d477" = 2
  constraints: 20 end point, 3 parallel, 3 perpendicular, 1 point on line, 1 vertical
  measures "d475" distance of L0.start L0.end
  measures "d476" distance of L0.end L1.end
  measures "d477" distance of L4.end L3.end
extrude "Extrusion69" add sketch "Sketch69" along normal blind 25
chamfer "Chamfer4" distance 18 distance2 25 1 edges at (75, 40, -24) measured on face at (55.6667, 40, -7.6667)
chamfer "Chamfer5" distance 18 distance2 25 1 edges at (75, 40, 24) measured on face at (55.6667, 40, -7.6667)
sketch "Sketch70" plane through (57, 15, 23) normal (1, 0, 0) x (0, 0, -1)
  line L0 (0, 0) -> (0, 25)
  line L1 (48, 25) -> (-2, 25)
  circle A0 centre (3, 21) radius 1.25
  circle A1 centre (3, 4) radius 1.25
  circle A2 centre (43, 4) radius 1.25
  circle A3 centre (43, 21) radius 1.25
  line L2 (8, 4) -> (8, 21)
  line L3 (8, 21) -> (38, 21)
  line L4 (38, 21) -> (38, 4)
  line L5 (38, 4) -> (8, 4)
  point P0 (23, -15)
  point P1 (-8.2218, -15)
  dimension "d488" = 2.5
  dimension "d489" = 2.5
  dimension "d490" = 2.5
  dimension "d491" = 5
  dimension "d492" = 30
  constraints: 12 end point, 4 centre point, 3 perpendicular
  measures "d488" diameter of A0
  measures "d489" diameter of A2
  measures "d490" diameter of A3
  measures "d491" distance of A1.centre L2.start
  measures "d492" distance of L2.end L3.end
extrude "Extrusion70" cut sketch "Sketch70" against normal blind 25
body "Solid1"
